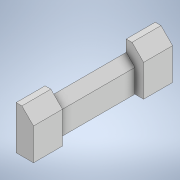
# Autodesk Inventor part: inside-join
Saved by Autodesk Inventor 2021 (Build 250183000, 183)
## iProperties
Created: 2020-12-08
Part Number: inside-join
Material: Generic
Document SubType Name: Modeling
Designer: Luke Kamols
Density: 1 g/cm^3
Appearance: Default
Author: Luke Kamols
Autodesk Inventor part; units mm, degrees
ref_plane "YZ Plane" through (0, 0, 0) normal (1, 0, 0) x (0, 1, 0)
ref_plane "XZ Plane" through (0, 0, 0) normal (0, 1, 0) x (-1, 0, 0)
ref_plane "XY Plane" through (0, 0, 0) normal (0, 0, 1) x (1, 0, 0)
sketch "Sketch1" plane through (0, 0, 0) normal (0, 0, 1) x (1, 0, 0)
  line L0 (0, 0) -> (0, 15)
  line L1 (0, 15) -> (2, 15)
  line L2 (0, 0) -> (6, 0)
  line L3 (6, 0) -> (6, 11)
  line L4 (6, 11) -> (2, 15)
  dimension "d0" = 15
  dimension "d1" = 2
  dimension "d2" = 6
  dimension "d3" = 11
  constraints: 10 end point, 2 perpendicular, 1 horizontal, 1 vertical
  measures "d0" distance of L0.start L0.end
  measures "d1" distance of L0.end L1.end
  measures "d2" distance of L0.start L2.end
  measures "d3" distance of L2.end L3.end
extrude "Extrusion1" add sketch "Sketch1" along normal blind 10
sketch "Sketch2" plane through (0, 0, 0) normal (0, 0, -1) x (-1, 0, 0)
  line L0 (0, 15) -> (0, 0) projected
  line L1 (0, 0) -> (-3, 0)
  line L2 (0, 0) -> (-6, 0) projected
  line L3 (-6, 11) -> (-2, 15) projected
  line L4 (0, 0) -> (3, 0)
  line L5 (0, 11) -> (-3, 8)
  line L6 (0, 11) -> (3, 8)
  line L7 (-3, 8) -> (-3, 0)
  line L8 (3, 8) -> (3, 0)
  constraints: 12 end point, 2 perpendicular, 1 midpoint, 1 point on line, 1 symmetric about line, 1 vertical
extrude "Extrusion2" add sketch "Sketch2" along normal blind 28
sketch "Sketch3" plane through (0, 0, -28) normal (0, 0, -1) x (-1, 0, 0)
  line L0 (0, 15) -> (0, 0) projected
  line L1 (0, 0) -> (-6, 0) projected
  line L2 (0, 0) -> (-6, 0)
  line L3 (-6, 0) -> (-6, 11) projected
  line L4 (-6, 0) -> (-6, 11)
  line L5 (-6, 11) -> (-2, 15) projected
  line L6 (-6, 11) -> (-2, 15)
  line L7 (-2, 15) -> (0, 15) projected
  line L8 (-2, 15) -> (0, 15)
  line L9 (0, 15) -> (0, 0)
  constraints: 10 end point, 3 collinear, 1 horizontal, 1 perpendicular
extrude "Extrusion3" add sketch "Sketch3" along normal blind 10
body "Solid1"
